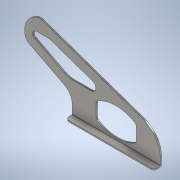
# Autodesk Inventor part: 0 零件
Saved by Autodesk Inventor 2020 (Build 240168000, 168)
## iProperties
Created: 2020-11-03
Part Number: 0 零件
Material: 不鏽鋼
Document SubType Name: Sheet Metal
Designer: p2013
Density: 8 g/cm^3
Appearance: 半拋光
Flat Pattern Width: 8.03676 cm
Flat Pattern Length: 20.0468 cm
Flat Pattern Area: 161.111 cm^2
Sheet Metal Rule: 預設 mm (_M)
Sheet Metal Width: 80.37 mm
Sheet Metal Length: 200.47 mm
Sheet Metal Area: 16111.15 mm^2
Author: p2013
Autodesk Inventor part; units mm, degrees
ref_plane "YZ Plane" through (0, 0, 0) normal (1, 0, 0) x (0, 1, 0)
ref_plane "XZ Plane" through (0, 0, 0) normal (0, 1, 0) x (-1, 0, 0)
ref_plane "XY Plane" through (0, 0, 0) normal (0, 0, 1) x (1, 0, 0)
sketch "草圖1" plane through (0, 0, 0) normal (0, 0, 1) x (1, 0, 0)
  line L0 (0, 0) -> (-40.5681, 0) construction
  line L1 (0, 0) -> (0, 45.2738) construction
  line L2 (-60, 18.7) -> (-21.9145, 18.7) construction
  line L3 (60, 18.1203) -> (60, 3.5)
  line L4 (56.5, 0) -> (-56.5, 0)
  line L5 (-60, 3.5) -> (-60, 18.7)
  line L6 (-87.6368, 8.7) -> (76.2221, 8.7)
  arc A0 (-60, 3.5) -> (-56.5, 0) centre (-56.5, 3.5) ccw
  arc A1 (56.5, 0) -> (60, 3.5) centre (56.5, 3.5) ccw
  arc A2 (-25, 17.157) -> (25, 17.157) centre (0, 60.4582) ccw
  line L7 (-27.5, 18.7) -> (27.5, 18.7) construction
  line L8 (16.8799, 18.7) -> (60, 18.7) construction
  line L9 (-60, 18.7) -> (-60, 20.4369)
  line L10 (-70.8518, 38.2221) -> (-119.0875, 63.0331)
  line L11 (-101.4762, 99.2795) -> (36.5219, 51.1695)
  arc A3 (-107.8929, 99.3362) -> (-124.1865, 69.3896) centre (-100.1179, 75.7) ccw
  line L12 (-104.2307, 100.2398) -> (-122.4731, 64.7746) construction
  line L13 (-92.566, 80.8091) -> (-108.8509, 80.8091)
  arc A4 (-89.2737, 80.2516) -> (-92.566, 80.8091) centre (-92.566, 70.8091) ccw
  line L14 (-32.7123, 60.5304) -> (-89.2737, 80.2516)
  arc A5 (-108.8509, 80.8091) -> (-110.452, 74.1968) centre (-108.8509, 77.3091) ccw
  line L15 (-110.452, 74.1968) -> (-70.3705, 53.5781)
  arc A6 (-70.3705, 53.5781) -> (-58.9345, 50.8091) centre (-58.9345, 75.8091) ccw
  line L16 (-58.9345, 50.8091) -> (-34.3585, 50.8091)
  arc A7 (-34.3585, 50.8091) -> (-32.7123, 60.5304) centre (-34.3585, 55.8091) ccw
  arc A8 (-88.7798, 81.668) -> (-92.566, 82.3091) centre (-92.566, 70.8091) ccw
  line L17 (-92.566, 82.3091) -> (-108.8509, 82.3091)
  arc A9 (-108.8509, 82.3091) -> (-111.1381, 72.8629) centre (-108.8509, 77.3091) ccw
  line L18 (-111.1381, 72.8629) -> (-71.0567, 52.2443)
  arc A10 (-71.0567, 52.2443) -> (-58.9345, 49.3091) centre (-58.9345, 75.8091) ccw
  line L19 (-58.9345, 49.3091) -> (-34.3585, 49.3091)
  arc A11 (-34.3585, 49.3091) -> (-32.2185, 61.9468) centre (-34.3585, 55.8091) ccw
  line L20 (-32.2185, 61.9468) -> (-88.7798, 81.668)
  arc A12 (-101.4762, 99.2795) -> (-107.8929, 99.3362) centre (-104.7682, 89.8369) ccw
  arc A13 (-124.1865, 69.3896) -> (-119.0875, 63.0331) centre (-114.5134, 71.9257) ccw
  arc A14 (25, 42.0013) -> (-25, 42.0013) centre (0, -1.3) ccw
  line L21 (-27.5, 37.6711) -> (-27.5, 21.4871)
  line L22 (27.5, 37.6711) -> (27.5, 21.4871)
  arc A15 (27.5, 37.6711) -> (25, 42.0013) centre (22.5, 37.6711) ccw
  arc A16 (25, 17.157) -> (27.5, 21.4871) centre (22.5, 21.4871) ccw
  arc A17 (-27.5, 21.4871) -> (-25, 17.157) centre (-22.5, 21.4871) ccw
  arc A18 (-25, 42.0013) -> (-27.5, 37.6711) centre (-22.5, 37.6711) ccw
  arc A19 (-60, 20.4369) -> (-70.8518, 38.2221) centre (-80, 20.4369) ccw
  arc A20 (60, 18.1203) -> (36.5219, 51.1695) centre (25, 18.1203) ccw
  point P0 (0, 0)
  point P1 (60, 42.9843)
  point P2 (-60, 40.3647)
  point P3 (-60, 32.6402)
  point P4 (27.5, 40.4582)
  point P5 (-27.5, 40.4582)
  point P6 (0, 18.7)
  dimension "d0" = 120
  dimension "d1" = 3.5
  dimension "d2" = 8.7
  dimension "d3" = 10
  dimension "d9" = 1.7582
  dimension "d12" = 117.22
  dimension "d14" = 8
  dimension "d16" = 24.8821
  dimension "d19" = 1.5
  dimension "d20" = 65
  dimension "d21" = 10
  dimension "d22" = 10
  dimension "d23" = 50
  dimension "d24" = 30
  dimension "d25" = 5
  dimension "d26" = 55
  dimension "d27" = 57
  dimension "d28" = 20
  dimension "d29" = 35
  dimension "d30" = 81.1369
  constraints: 49 point on circle, 46 end point, 21 centre point, 20 tangent, 17 point on line, 7 horizontal, 6 equal radius, 6 perpendicular, 4 parallel, 3 midpoint, 2 vertical, 2 vertical alignment, 27 other
  measures "d0" distance between parallel lines of L3 L5
  measures "d1" radius of A0
  measures "d2" distance between parallel lines of L6 L4
  measures "d3" distance between parallel lines of L6 L2
  measures "d9" distance edge to line of A2 L6
  measures "d12" angle of L9 L10
  measures "d14" angle of L10 L11
  measures "d16" radius of A3
  measures "d19" distance between parallel lines of L18 L15
  measures "d21" radius of A12
  measures "d22" distance edge to line of A3 L12
  measures "d23" radius of A14
  measures "d24" distance edge to line of A14 L7
  measures "d25" radius of A15
  measures "d26" distance between parallel lines of L22 L21
  measures "d27" distance from line of L7 A3.centre
  measures "d28" radius of A19
  measures "d29" radius of A20
extrude "擠出1" add sketch "草圖1" against normal blind 2 contours L3 L6 L5 L9 A19 L10 A13 A3 A12 L11 A20 | L3 A1 L4 A0 L5 L6
bend part "折彎零件1" radius 0.4 angle 85 line through (-87.6368, 8.7, 0) along (1, 0, 0) centre toward (0, 0, 1) moving side (0, -1, 0) both sides no
equation "\"折彎半徑\" = 厚度"
equation "\"折彎離隙寬度\" = 厚度"
equation "\"折彎離隙深度\" = 0.5 * 厚度"
equation "\"轉角離隙大小\" = 4 * 厚度"
equation "\"最小剩餘\" = 2 * 厚度"
equation "\"轉移半徑\" = 折彎半徑"
equation "\"Jacobi半徑大小\" = 折彎半徑"
equation "\"間隙大小\" = 厚度"
equation "\"厚度\" = 2"
